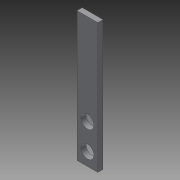
# Autodesk Inventor part: Y_Rail_Limit_Rod-SquareBar-Rev3
Saved by Autodesk Inventor 2015 (Build 190159000, 159)
## iProperties
Created: 2017-01-12
Part Number: Y_Rail_Limit_Rod-SquareBar-Rev3
Material: Generic
Document SubType Name: Modeling
Designer: Guy
Density: 1 g/cm^3
Appearance: Default
Author: Guy
Autodesk Inventor part; units mm, degrees
ref_plane "YZ Plane" through (0, 0, 0) normal (1, 0, 0) x (0, 1, 0)
ref_plane "XZ Plane" through (0, 0, 0) normal (0, 1, 0) x (-1, 0, 0)
ref_plane "XY Plane" through (0, 0, 0) normal (0, 0, 1) x (1, 0, 0)
sketch "Sketch1" plane through (0, 0, 0) normal (0, 0, 1) x (1, 0, 0)
  line L0 (0, 0) -> (8, 0)
  line L1 (8, 0) -> (8, 2)
  line L2 (8, 2) -> (0, 2)
  line L3 (0, 2) -> (0, 0)
  dimension "d0" = 8
  dimension "d1" = 2
  constraints: 8 end point, 2 parallel, 1 horizontal, 1 perpendicular
  measures "d0" distance of L2.end L1.end
  measures "d1" distance between parallel lines of L0 L2
extrude "Extrusion1" add sketch "Sketch1" along normal blind 50
sketch "Sketch2" plane through (0, 0, 0) normal (0, -1, 0) x (1, 0, 0)
  circle A0 centre (4, 5) radius 2.5
  circle A1 centre (4, 15) radius 2.5
  line L0 (0, 0) -> (8, 0) projected
  line L1 (8, 0) -> (8, 50) projected
  line L2 (0, 50) -> (8, 50) projected
  line L3 (0, 0) -> (0, 50) projected
  dimension "d4" = 5
  dimension "d5" = 5
  dimension "d6" = 5
  dimension "d7" = 10
  dimension "d8" = 4
  dimension "d9" = 4
  constraints: 2 centre point
  measures "d4" diameter of A0
  measures "d5" diameter of A1
  measures "d6" distance from line of L0 A0.centre
  measures "d7" distance of A0.centre A1.centre
  measures "d8" distance from line of L1 A0.centre
  measures "d9" distance from line of L1 A1.centre
extrude "Extrusion2" cut sketch "Sketch2" against normal up to next contours A0 | A1
body "Solid1"
